Autodesk Fusion 360 part; units mm, degrees
note: some values were not read from the file. Set by a fixed rule: which sketch regions a step uses.
(part 20 of 20)
  spline S115 degree 5 poles (0.9213, 29.0307) (0.9213, 29.0307) (0.9213, 29.0309) (0.9213, 29.0313) (0.9213, 29.0318) (0.9213, 29.0325) (0.9213, 29.0334) (0.9214, 29.0344) (0.9214, 29.0355) (0.9214, 29.0367) (0.9214, 29.038) (0.9214, 29.0394) (0.9214, 29.0409) (0.9214, 29.0425) (0.9214, 29.0443) (0.9214, 29.0461) (0.9214, 29.0481) (0.9214, 29.0501) (0.9214, 29.0522) (0.9214, 29.0545) (0.9214, 29.0568) (0.9213, 29.0592) (0.9213, 29.0618) (0.9212, 29.0644) (0.9212, 29.0671) (0.9211, 29.0699) (0.9211, 29.0728) (0.921, 29.0758) (0.9209, 29.0788) (0.9208, 29.082) (0.9208, 29.0852) (0.9206, 29.0886) (0.9205, 29.092) (0.9204, 29.0955) (0.9203, 29.0991) (0.9201, 29.1028) (0.92, 29.1065) (0.9198, 29.1103) (0.9197, 29.1143) (0.9195, 29.1183) (0.9193, 29.1223) (0.9191, 29.1265) (0.9189, 29.1307) (0.9186, 29.135) (0.9184, 29.1394) (0.9182, 29.1439) (0.9179, 29.1484) (0.9176, 29.153) (0.9173, 29.1577) (0.917, 29.1624) (0.9167, 29.1673) (0.9164, 29.1722) (0.9161, 29.1771) (0.9157, 29.1822) (0.9153, 29.1873) (0.915, 29.1925) (0.9146, 29.1977) (0.9141, 29.203) (0.9137, 29.2084) (0.9133, 29.2139) (0.9128, 29.2194) (0.9124, 29.225) (0.9119, 29.2306) (0.9114, 29.2363) (0.9109, 29.2421) (0.9103, 29.248) (0.9098, 29.2539) (0.9092, 29.2599) (0.9087, 29.2659) (0.9081, 29.272) (0.9075, 29.2781) (0.9068, 29.2844) (0.9062, 29.2906) (0.9055, 29.297) (0.9049, 29.3034) (0.9042, 29.3099) (0.9035, 29.3164) (0.9027, 29.323) (0.902, 29.3296) (0.9012, 29.3363) (0.9005, 29.343) (0.8997, 29.3498) (0.8989, 29.3567) (0.898, 29.3636) (0.8972, 29.3706) (0.8963, 29.3777) (0.8954, 29.3847) (0.8945, 29.3919) (0.8936, 29.3991) (0.8927, 29.4063) (0.8917, 29.4137) (0.8907, 29.421) (0.8897, 29.4284) (0.8887, 29.4359) (0.8877, 29.4434) (0.8866, 29.451) (0.8856, 29.4586) (0.8845, 29.4663) (0.8834, 29.474) (0.8822, 29.4818) (0.8811, 29.4896) (0.8799, 29.4975) (0.8787, 29.5054) (0.8775, 29.5134) (0.8763, 29.5214) (0.875, 29.5295) (0.8738, 29.5376) (0.8725, 29.5458) (0.8712, 29.554) (0.8698, 29.5623) (0.8685, 29.5706) (0.8671, 29.5789) (0.8657, 29.5873) (0.8643, 29.5958) (0.8629, 29.6043) (0.8614, 29.6128) (0.86, 29.6214) (0.8585, 29.6301) (0.8569, 29.6388) (0.8554, 29.6475) (0.8538, 29.6563) (0.8523, 29.6651) (0.8507, 29.6739) (0.849, 29.6828) (0.8474, 29.6918) (0.8457, 29.7008) (0.844, 29.7098) (0.8423, 29.7189) (0.8406, 29.728) (0.8388, 29.7372) (0.8371, 29.7464) (0.8353, 29.7556) (0.8334, 29.7649) (0.8316, 29.7742) (0.8297, 29.7836) (0.8279, 29.793) (0.8259, 29.8025) (0.824, 29.812) (0.8221, 29.8215) (0.8201, 29.8311) (0.8181, 29.8407) (0.8161, 29.8503) (0.814, 29.86) (0.812, 29.8697) (0.8099, 29.8795) (0.8078, 29.8893) (0.8056, 29.8992) (0.8035, 29.909) (0.8013, 29.919) (0.7991, 29.9289) (0.7969, 29.9389) (0.7946, 29.949) (0.7923, 29.959) (0.79, 29.9691) (0.7877, 29.9793) (0.7854, 29.9895) (0.783, 29.9997) (0.7806, 30.0099) (0.7782, 30.0202) (0.7758, 30.0306) (0.7733, 30.0409) (0.7708, 30.0513) (0.7683, 30.0618) (0.7658, 30.0722) (0.7632, 30.0827) (0.7606, 30.0933) (0.758, 30.1038) (0.7554, 30.1145) (0.7528, 30.1251) (0.7501, 30.1358) (0.7474, 30.1465) (0.7447, 30.1572) (0.7419, 30.168) (0.7391, 30.1788) (0.7364, 30.1897) (0.7335, 30.2005) (0.7307, 30.2114) (0.7278, 30.2224) (0.7249, 30.2334) (0.722, 30.2444) (0.7191, 30.2554) (0.7161, 30.2665) (0.7131, 30.2776) (0.7101, 30.2887) (0.7071, 30.2999) (0.704, 30.3111) (0.7009, 30.3223) (0.6978, 30.3336) (0.6947, 30.3448) (0.6915, 30.3562) (0.6883, 30.3675) (0.6851, 30.3789) (0.6819, 30.3903) (0.6786, 30.4017) (0.6753, 30.4132) (0.672, 30.4247) (0.6687, 30.4362) (0.6653, 30.4478) (0.6619, 30.4594) (0.6585, 30.471) (0.6551, 30.4827) (0.6516, 30.4943) (0.6481, 30.506) (0.6446, 30.5178) (0.6411, 30.5295) (0.6375, 30.5413) (0.6339, 30.5531) (0.6303, 30.565) (0.6267, 30.5769) (0.623, 30.5888) (0.6193, 30.6007) (0.6156, 30.6126) (0.6118, 30.6246) (0.6081, 30.6366) (0.6043, 30.6487) (0.6005, 30.6607) (0.5966, 30.6728) (0.5927, 30.685) (0.5889, 30.6971) (0.5849, 30.7093) (0.581, 30.7215) (0.577, 30.7337) (0.573, 30.7459) (0.569, 30.7582) (0.5649, 30.7705) (0.5609, 30.7828) (0.5568, 30.7952) (0.5526, 30.8076) (0.5485, 30.82) (0.5443, 30.8324) (0.5401, 30.8448) (0.5359, 30.8573) (0.5316, 30.8698) (0.5273, 30.8823) (0.523, 30.8949) (0.5187, 30.9075) (0.5143, 30.9201) (0.5099, 30.9327) (0.5055, 30.9453) (0.5011, 30.958) (0.4966, 30.9707) (0.493, 30.9809) (0.4903, 30.9885) (0.4885, 30.9936) (0.4876, 30.9962) knots 0 0 0 0 0 0 0.00416667 0.00833333 0.0125 0.01666667 0.02083333 0.025 0.02916667 0.03333333 0.0375 0.04166667 0.04583333 0.05 0.05416667 0.05833333 0.0625 0.06666667 0.07083333 0.075 0.07916667 0.08333333 0.0875 0.09166667 0.09583333 0.1 0.10416667 0.10833333 0.1125 0.11666667 0.12083333 0.125 0.12916667 0.13333333 0.1375 0.14166667 0.14583333 0.15 0.15416667 0.15833333 0.1625 0.16666667 0.17083333 0.175 0.17916667 0.18333333 0.1875 0.19166667 0.19583333 0.2 0.20416667 0.20833333 0.2125 0.21666667 0.22083333 0.225 0.22916667 0.23333333 0.2375 0.24166667 0.24583333 0.25 0.25416667 0.25833333 0.2625 0.26666667 0.27083333 0.275 0.27916667 0.28333333 0.2875 0.29166667 0.29583333 0.3 0.30416667 0.30833333 0.3125 0.31666667 0.32083333 0.325 0.32916667 0.33333333 0.3375 0.34166667 0.34583333 0.35 0.35416667 0.35833333 0.3625 0.36666667 0.37083333 0.375 0.37916667 0.38333333 0.3875 0.39166667 0.39583333 0.4 0.40416667 0.40833333 0.4125 0.41666667 0.42083333 0.425 0.42916667 0.43333333 0.4375 0.44166667 0.44583333 0.45 0.45416667 0.45833333 0.4625 0.46666667 0.47083333 0.475 0.47916667 0.48333333 0.4875 0.49166667 0.49583333 0.5 0.50416667 0.50833333 0.5125 0.51666667 0.52083333 0.525 0.52916667 0.53333333 0.5375 0.54166667 0.54583333 0.55 0.55416667 0.55833333 0.5625 0.56666667 0.57083333 0.575 0.57916667 0.58333333 0.5875 0.59166667 0.59583333 0.6 0.60416667 0.60833333 0.6125 0.61666667 0.62083333 0.625 0.62916667 0.63333333 0.6375 0.64166667 0.64583333 0.65 0.65416667 0.65833333 0.6625 0.66666667 0.67083333 0.675 0.67916667 0.68333333 0.6875 0.69166667 0.69583333 0.7 0.70416667 0.70833333 0.7125 0.71666667 0.72083333 0.725 0.72916667 0.73333333 0.7375 0.74166667 0.74583333 0.75 0.75416667 0.75833333 0.7625 0.76666667 0.77083333 0.775 0.77916667 0.78333333 0.7875 0.79166667 0.79583333 0.8 0.80416667 0.80833333 0.8125 0.81666667 0.82083333 0.825 0.82916667 0.83333333 0.8375 0.84166667 0.84583333 0.85 0.85416667 0.85833333 0.8625 0.86666667 0.87083333 0.875 0.87916667 0.88333333 0.8875 0.89166667 0.89583333 0.9 0.90416667 0.90833333 0.9125 0.91666667 0.92083333 0.925 0.92916667 0.93333333 0.9375 0.94166667 0.94583333 0.95 0.95416667 0.95833333 0.9625 0.96666667 0.97083333 0.975 0.97916667 0.98333333 0.9875 0.99166667 0.99583333 1 1 1 1 1 1
  line L225 (-24.6799, 15.3128) -> (-24.6806, 15.3132)
  line L226 (0.9119, 28.7355) -> (0.9213, 29.0298)
  line L227 (0.9213, 29.0298) -> (0.9213, 29.0307)
  line L228 (-25.6019, 13.7175) -> (-25.6012, 13.7171)
  line L229 (-24.0271, 16.318) -> (-23.7836, 16.1526)
  arc A119 (2.0967, 28.6734) -> (0.9119, 28.7355) centre (0, 0) ccw
  arc A120 (-26.5997, 15.9204) -> (-27.0873, 15.0758) centre (0, 0) ccw
  line L230 (-27.8937, 8.0945) -> (-27.6109, 8.0125)
  arc A121 (-28.2972, 5.0824) -> (-28.4828, 3.9106) centre (0, 0) ccw
  spline S116 degree 5 poles (-28.2047, 6.937) (-28.2048, 6.937) (-28.205, 6.937) (-28.2053, 6.9371) (-28.2058, 6.9372) (-28.2065, 6.9374) (-28.2074, 6.9376) (-28.2083, 6.9378) (-28.2094, 6.9381) (-28.2106, 6.9383) (-28.2118, 6.9386) (-28.2132, 6.9389) (-28.2147, 6.9392) (-28.2163, 6.9396) (-28.218, 6.9399) (-28.2198, 6.9403) (-28.2217, 6.9407) (-28.2237, 6.9411) (-28.2258, 6.9416) (-28.228, 6.942) (-28.2303, 6.9425) (-28.2327, 6.9429) (-28.2351, 6.9434) (-28.2377, 6.9439) (-28.2404, 6.9445) (-28.2431, 6.945) (-28.246, 6.9455) (-28.2489, 6.9461) (-28.2519, 6.9466) (-28.255, 6.9472) (-28.2582, 6.9478) (-28.2615, 6.9484) (-28.2649, 6.949) (-28.2683, 6.9496) (-28.2719, 6.9502) (-28.2755, 6.9508) (-28.2792, 6.9515) (-28.283, 6.9521) (-28.2868, 6.9528) (-28.2908, 6.9534) (-28.2948, 6.9541) (-28.2989, 6.9547) (-28.3031, 6.9554) (-28.3074, 6.9561) (-28.3117, 6.9568) (-28.3161, 6.9574) (-28.3206, 6.9581) (-28.3252, 6.9588) (-28.3298, 6.9595) (-28.3345, 6.9602) (-28.3393, 6.9609) (-28.3442, 6.9616) (-28.3491, 6.9623) (-28.3541, 6.963) (-28.3592, 6.9637) (-28.3643, 6.9644) (-28.3695, 6.9651) (-28.3748, 6.9658) (-28.3802, 6.9665) (-28.3856, 6.9672) (-28.3911, 6.9679) (-28.3966, 6.9686) (-28.4023, 6.9693) (-28.408, 6.97) (-28.4137, 6.9707) (-28.4196, 6.9714) (-28.4255, 6.9721) (-28.4314, 6.9728) (-28.4374, 6.9735) (-28.4435, 6.9742) (-28.4497, 6.9749) (-28.4559, 6.9756) (-28.4622, 6.9763) (-28.4685, 6.9769) (-28.4749, 6.9776) (-28.4814, 6.9783) (-28.4879, 6.9789) (-28.4945, 6.9796) (-28.5011, 6.9803) (-28.5078, 6.9809) (-28.5146, 6.9816) (-28.5214, 6.9822) (-28.5283, 6.9828) (-28.5353, 6.9835) (-28.5423, 6.9841) (-28.5493, 6.9847) (-28.5564, 6.9853) (-28.5636, 6.9859) (-28.5709, 6.9865) (-28.5781, 6.9871) (-28.5855, 6.9877) (-28.5929, 6.9882) (-28.6004, 6.9888) (-28.6079, 6.9894) (-28.6154, 6.9899) (-28.6231, 6.9905) (-28.6307, 6.991) (-28.6385, 6.9915) (-28.6463, 6.9921) (-28.6541, 6.9926) (-28.662, 6.9931) (-28.67, 6.9936) (-28.678, 6.994) (-28.686, 6.9945) (-28.6941, 6.995) (-28.7023, 6.9954) (-28.7105, 6.9959) (-28.7187, 6.9963) (-28.727, 6.9968) (-28.7354, 6.9972) (-28.7438, 6.9976) (-28.7523, 6.998) (-28.7608, 6.9984) (-28.7694, 6.9987) (-28.778, 6.9991) (-28.7866, 6.9995) (-28.7953, 6.9998) (-28.8041, 7.0001) (-28.8129, 7.0005) (-28.8218, 7.0008) (-28.8307, 7.0011) (-28.8396, 7.0014) (-28.8486, 7.0016) (-28.8577, 7.0019) (-28.8668, 7.0021) (-28.8759, 7.0024) (-28.8851, 7.0026) (-28.8943, 7.0028) (-28.9036, 7.003) (-28.9129, 7.0032) (-28.9223, 7.0034) (-28.9317, 7.0036) (-28.9412, 7.0037) (-28.9507, 7.0038) (-28.9602, 7.004) (-28.9698, 7.0041) (-28.9795, 7.0042) (-28.9892, 7.0043) (-28.9989, 7.0043) (-29.0087, 7.0044) (-29.0185, 7.0044) (-29.0284, 7.0045) (-29.0383, 7.0045) (-29.0482, 7.0045) (-29.0582, 7.0045) (-29.0682, 7.0044) (-29.0783, 7.0044) (-29.0884, 7.0043) (-29.0986, 7.0043) (-29.1088, 7.0042) (-29.119, 7.0041) (-29.1293, 7.004) (-29.1396, 7.0038) (-29.15, 7.0037) (-29.1604, 7.0035) (-29.1708, 7.0034) (-29.1813, 7.0032) (-29.1919, 7.003) (-29.2024, 7.0028) (-29.213, 7.0025) (-29.2237, 7.0023) (-29.2344, 7.002) (-29.2451, 7.0017) (-29.2559, 7.0014) (-29.2667, 7.0011) (-29.2775, 7.0008) (-29.2884, 7.0004) (-29.2993, 7.0001) (-29.3103, 6.9997) (-29.3213, 6.9993) (-29.3323, 6.9989) (-29.3434, 6.9984) (-29.3545, 6.998) (-29.3657, 6.9975) (-29.3768, 6.997) (-29.3881, 6.9965) (-29.3993, 6.996) (-29.4106, 6.9955) (-29.422, 6.995) (-29.4333, 6.9944) (-29.4447, 6.9938) (-29.4562, 6.9932) (-29.4677, 6.9926) (-29.4792, 6.992) (-29.4907, 6.9913) (-29.5023, 6.9906) (-29.514, 6.99) (-29.5256, 6.9892) (-29.5373, 6.9885) (-29.549, 6.9878) (-29.5608, 6.987) (-29.5726, 6.9863) (-29.5844, 6.9855) (-29.5963, 6.9846) (-29.6082, 6.9838) (-29.6201, 6.983) (-29.6321, 6.9821) (-29.6441, 6.9812) (-29.6562, 6.9803) (-29.6682, 6.9794) (-29.6803, 6.9784) (-29.6925, 6.9775) (-29.7047, 6.9765) (-29.7169, 6.9755) (-29.7291, 6.9745) (-29.7414, 6.9735) (-29.7537, 6.9724) (-29.766, 6.9713) (-29.7784, 6.9702) (-29.7908, 6.9691) (-29.8032, 6.968) (-29.8157, 6.9669) (-29.8282, 6.9657) (-29.8407, 6.9645) (-29.8533, 6.9633) (-29.8659, 6.9621) (-29.8785, 6.9608) (-29.8912, 6.9596) (-29.9039, 6.9583) (-29.9166, 6.957) (-29.9293, 6.9556) (-29.9421, 6.9543) (-29.9549, 6.9529) (-29.9678, 6.9516) (-29.9806, 6.9501) (-29.9935, 6.9487) (-30.0065, 6.9473) (-30.0194, 6.9458) (-30.0324, 6.9443) (-30.0455, 6.9428) (-30.0585, 6.9413) (-30.0716, 6.9398) (-30.0847, 6.9382) (-30.0979, 6.9366) (-30.111, 6.935) (-30.1242, 6.9334) (-30.1375, 6.9317) (-30.1507, 6.9301) (-30.164, 6.9284) (-30.1773, 6.9267) (-30.1907, 6.925) (-30.2014, 6.9236) (-30.2094, 6.9225) (-30.2148, 6.9218) (-30.2174, 6.9214) knots 0 0 0 0 0 0 0.00416667 0.00833333 0.0125 0.01666667 0.02083333 0.025 0.02916667 0.03333333 0.0375 0.04166667 0.04583333 0.05 0.05416667 0.05833333 0.0625 0.06666667 0.07083333 0.075 0.07916667 0.08333333 0.0875 0.09166667 0.09583333 0.1 0.10416667 0.10833333 0.1125 0.11666667 0.12083333 0.125 0.12916667 0.13333333 0.1375 0.14166667 0.14583333 0.15 0.15416667 0.15833333 0.1625 0.16666667 0.17083333 0.175 0.17916667 0.18333333 0.1875 0.19166667 0.19583333 0.2 0.20416667 0.20833333 0.2125 0.21666667 0.22083333 0.225 0.22916667 0.23333333 0.2375 0.24166667 0.24583333 0.25 0.25416667 0.25833333 0.2625 0.26666667 0.27083333 0.275 0.27916667 0.28333333 0.2875 0.29166667 0.29583333 0.3 0.30416667 0.30833333 0.3125 0.31666667 0.32083333 0.325 0.32916667 0.33333333 0.3375 0.34166667 0.34583333 0.35 0.35416667 0.35833333 0.3625 0.36666667 0.37083333 0.375 0.37916667 0.38333333 0.3875 0.39166667 0.39583333 0.4 0.40416667 0.40833333 0.4125 0.41666667 0.42083333 0.425 0.42916667 0.43333333 0.4375 0.44166667 0.44583333 0.45 0.45416667 0.45833333 0.4625 0.46666667 0.47083333 0.475 0.47916667 0.48333333 0.4875 0.49166667 0.49583333 0.5 0.50416667 0.50833333 0.5125 0.51666667 0.52083333 0.525 0.52916667 0.53333333 0.5375 0.54166667 0.54583333 0.55 0.55416667 0.55833333 0.5625 0.56666667 0.57083333 0.575 0.57916667 0.58333333 0.5875 0.59166667 0.59583333 0.6 0.60416667 0.60833333 0.6125 0.61666667 0.62083333 0.625 0.62916667 0.63333333 0.6375 0.64166667 0.64583333 0.65 0.65416667 0.65833333 0.6625 0.66666667 0.67083333 0.675 0.67916667 0.68333333 0.6875 0.69166667 0.69583333 0.7 0.70416667 0.70833333 0.7125 0.71666667 0.72083333 0.725 0.72916667 0.73333333 0.7375 0.74166667 0.74583333 0.75 0.75416667 0.75833333 0.7625 0.76666667 0.77083333 0.775 0.77916667 0.78333333 0.7875 0.79166667 0.79583333 0.8 0.80416667 0.80833333 0.8125 0.81666667 0.82083333 0.825 0.82916667 0.83333333 0.8375 0.84166667 0.84583333 0.85 0.85416667 0.85833333 0.8625 0.86666667 0.87083333 0.875 0.87916667 0.88333333 0.8875 0.89166667 0.89583333 0.9 0.90416667 0.90833333 0.9125 0.91666667 0.92083333 0.925 0.92916667 0.93333333 0.9375 0.94166667 0.94583333 0.95 0.95416667 0.95833333 0.9625 0.96666667 0.97083333 0.975 0.97916667 0.98333333 0.9875 0.99166667 0.99583333 1 1 1 1 1 1
  line L231 (-28.587, 5.1345) -> (-28.2972, 5.0824)
  line L232 (-28.5878, 5.1346) -> (-28.587, 5.1345)
  spline S117 degree 5 poles (-30.4202, 5.9675) (-30.4179, 5.9661) (-30.4133, 5.9633) (-30.4064, 5.959) (-30.3972, 5.9534) (-30.3857, 5.9464) (-30.3742, 5.9394) (-30.3628, 5.9325) (-30.3513, 5.9255) (-30.3399, 5.9187) (-30.3285, 5.9118) (-30.3171, 5.905) (-30.3058, 5.8982) (-30.2944, 5.8914) (-30.2831, 5.8847) (-30.2718, 5.878) (-30.2605, 5.8713) (-30.2492, 5.8647) (-30.238, 5.8581) (-30.2268, 5.8515) (-30.2156, 5.8449) (-30.2044, 5.8384) (-30.1932, 5.8319) (-30.1821, 5.8255) (-30.1709, 5.8191) (-30.1598, 5.8127) (-30.1487, 5.8063) (-30.1377, 5.8) (-30.1266, 5.7937) (-30.1156, 5.7874) (-30.1046, 5.7811) (-30.0936, 5.7749) (-30.0826, 5.7688) (-30.0717, 5.7626) (-30.0608, 5.7565) (-30.0499, 5.7504) (-30.039, 5.7443) (-30.0281, 5.7383) (-30.0173, 5.7323) (-30.0065, 5.7263) (-29.9957, 5.7204) (-29.9849, 5.7145) (-29.9742, 5.7086) (-29.9634, 5.7028) (-29.9527, 5.697) (-29.9421, 5.6912) (-29.9314, 5.6854) (-29.9208, 5.6797) (-29.9102, 5.674) (-29.8996, 5.6683) (-29.889, 5.6627) (-29.8785, 5.6571) (-29.868, 5.6515) (-29.8575, 5.646) (-29.847, 5.6405) (-29.8366, 5.635) (-29.8262, 5.6296) (-29.8158, 5.6242) (-29.8054, 5.6188) (-29.7951, 5.6134) (-29.7847, 5.6081) (-29.7745, 5.6028) (-29.7642, 5.5975) (-29.754, 5.5923) (-29.7437, 5.5871) (-29.7336, 5.5819) (-29.7234, 5.5768) (-29.7133, 5.5717) (-29.7032, 5.5666) (-29.6931, 5.5615) (-29.683, 5.5565) (-29.673, 5.5515) (-29.663, 5.5466) (-29.653, 5.5416) (-29.6431, 5.5367) (-29.6332, 5.5319) (-29.6233, 5.527) (-29.6134, 5.5222) (-29.6036, 5.5175) (-29.5938, 5.5127) (-29.584, 5.508) (-29.5743, 5.5033) (-29.5646, 5.4987) (-29.5549, 5.494) (-29.5452, 5.4895) (-29.5356, 5.4849) (-29.526, 5.4804) (-29.5165, 5.4759) (-29.5069, 5.4714) (-29.4974, 5.467) (-29.4879, 5.4625) (-29.4785, 5.4582) (-29.4691, 5.4538) (-29.4597, 5.4495) (-29.4504, 5.4452) (-29.441, 5.441) (-29.4318, 5.4367) (-29.4225, 5.4325) (-29.4133, 5.4284) (-29.4041, 5.4242) (-29.395, 5.4201) (-29.3858, 5.4161) (-29.3767, 5.412) (-29.3677, 5.408) (-29.3587, 5.404) (-29.3497, 5.4001) (-29.3407, 5.3961) (-29.3318, 5.3922) (-29.3229, 5.3884) (-29.3141, 5.3846) (-29.3053, 5.3807) (-29.2965, 5.377) (-29.2878, 5.3732) (-29.279, 5.3695) (-29.2704, 5.3658) (-29.2617, 5.3622) (-29.2531, 5.3586) (-29.2446, 5.355) (-29.2361, 5.3514) (-29.2276, 5.3479) (-29.2191, 5.3444) (-29.2107, 5.3409) (-29.2023, 5.3375) (-29.194, 5.3341) (-29.1857, 5.3307) (-29.1775, 5.3273) (-29.1692, 5.324) (-29.1611, 5.3207) (-29.1529, 5.3175) (-29.1448, 5.3143) (-29.1368, 5.3111) (-29.1288, 5.3079) (-29.1208, 5.3047) (-29.1129, 5.3016) (-29.105, 5.2986) (-29.0971, 5.2955) (-29.0893, 5.2925) (-29.0815, 5.2895) (-29.0738, 5.2865) (-29.0661, 5.2836) (-29.0585, 5.2807) (-29.0509, 5.2778) (-29.0433, 5.275) (-29.0358, 5.2722) (-29.0284, 5.2694) (-29.021, 5.2666) (-29.0136, 5.2639) (-29.0063, 5.2612) (-28.999, 5.2586) (-28.9918, 5.2559) (-28.9846, 5.2533) (-28.9774, 5.2508) (-28.9703, 5.2482) (-28.9633, 5.2457) (-28.9563, 5.2432) (-28.9493, 5.2408) (-28.9424, 5.2383) (-28.9356, 5.2359) (-28.9288, 5.2336) (-28.922, 5.2312) (-28.9153, 5.2289) (-28.9087, 5.2266) (-28.9021, 5.2244) (-28.8955, 5.2222) (-28.889, 5.22) (-28.8826, 5.2178) (-28.8762, 5.2157) (-28.8699, 5.2136) (-28.8636, 5.2115) (-28.8573, 5.2094) (-28.8512, 5.2074) (-28.8451, 5.2054) (-28.839, 5.2035) (-28.833, 5.2015) (-28.827, 5.1996) (-28.8211, 5.1978) (-28.8153, 5.1959) (-28.8095, 5.1941) (-28.8038, 5.1923) (-28.7981, 5.1905) (-28.7925, 5.1888) (-28.7869, 5.1871) (-28.7815, 5.1854) (-28.776, 5.1838) (-28.7707, 5.1822) (-28.7654, 5.1806) (-28.7601, 5.179) (-28.7549, 5.1775) (-28.7498, 5.176) (-28.7448, 5.1745) (-28.7398, 5.173) (-28.7349, 5.1716) (-28.73, 5.1702) (-28.7252, 5.1689) (-28.7205, 5.1675) (-28.7158, 5.1662) (-28.7112, 5.1649) (-28.7067, 5.1637) (-28.7023, 5.1625) (-28.6979, 5.1613) (-28.6936, 5.1601) (-28.6893, 5.1589) (-28.6852, 5.1578) (-28.6811, 5.1567) (-28.6771, 5.1557) (-28.6731, 5.1546) (-28.6693, 5.1536) (-28.6655, 5.1527) (-28.6617, 5.1517) (-28.6581, 5.1508) (-28.6545, 5.1499) (-28.6511, 5.149) (-28.6477, 5.1481) (-28.6443, 5.1473) (-28.6411, 5.1465) (-28.6379, 5.1458) (-28.6349, 5.145) (-28.6319, 5.1443) (-28.629, 5.1436) (-28.6262, 5.143) (-28.6234, 5.1423) (-28.6208, 5.1417) (-28.6182, 5.1411) (-28.6158, 5.1406) (-28.6134, 5.14) (-28.6111, 5.1395) (-28.6089, 5.139) (-28.6069, 5.1386) (-28.6049, 5.1381) (-28.603, 5.1377) (-28.6012, 5.1374) (-28.5995, 5.137) (-28.5979, 5.1367) (-28.5964, 5.1363) (-28.595, 5.1361) (-28.5937, 5.1358) (-28.5925, 5.1356) (-28.5915, 5.1354) (-28.5905, 5.1352) (-28.5896, 5.135) (-28.5889, 5.1349) (-28.5884, 5.1348) (-28.5881, 5.1347) (-28.5879, 5.1347) (-28.5878, 5.1346) knots -1 -1 -1 -1 -1 -1 -0.99583333 -0.99166667 -0.9875 -0.98333333 -0.97916667 -0.975 -0.97083333 -0.96666667 -0.9625 -0.95833333 -0.95416667 -0.95 -0.94583333 -0.94166667 -0.9375 -0.93333333 -0.92916667 -0.925 -0.92083333 -0.91666667 -0.9125 -0.90833333 -0.90416667 -0.9 -0.89583333 -0.89166667 -0.8875 -0.88333333 -0.87916667 -0.875 -0.87083333 -0.86666667 -0.8625 -0.85833333 -0.85416667 -0.85 -0.84583333 -0.84166667 -0.8375 -0.83333333 -0.82916667 -0.825 -0.82083333 -0.81666667 -0.8125 -0.80833333 -0.80416667 -0.8 -0.79583333 -0.79166667 -0.7875 -0.78333333 -0.77916667 -0.775 -0.77083333 -0.76666667 -0.7625 -0.75833333 -0.75416667 -0.75 -0.74583333 -0.74166667 -0.7375 -0.73333333 -0.72916667 -0.725 -0.72083333 -0.71666667 -0.7125 -0.70833333 -0.70416667 -0.7 -0.69583333 -0.69166667 -0.6875 -0.68333333 -0.67916667 -0.675 -0.67083333 -0.66666667 -0.6625 -0.65833333 -0.65416667 -0.65 -0.64583333 -0.64166667 -0.6375 -0.63333333 -0.62916667 -0.625 -0.62083333 -0.61666667 -0.6125 -0.60833333 -0.60416667 -0.6 -0.59583333 -0.59166667 -0.5875 -0.58333333 -0.57916667 -0.575 -0.57083333 -0.56666667 -0.5625 -0.55833333 -0.55416667 -0.55 -0.54583333 -0.54166667 -0.5375 -0.53333333 -0.52916667 -0.525 -0.52083333 -0.51666667 -0.5125 -0.50833333 -0.50416667 -0.5 -0.49583333 -0.49166667 -0.4875 -0.48333333 -0.47916667 -0.475 -0.47083333 -0.46666667 -0.4625 -0.45833333 -0.45416667 -0.45 -0.44583333 -0.44166667 -0.4375 -0.43333333 -0.42916667 -0.425 -0.42083333 -0.41666667 -0.4125 -0.40833333 -0.40416667 -0.4 -0.39583333 -0.39166667 -0.3875 -0.38333333 -0.37916667 -0.375 -0.37083333 -0.36666667 -0.3625 -0.35833333 -0.35416667 -0.35 -0.34583333 -0.34166667 -0.3375 -0.33333333 -0.32916667 -0.325 -0.32083333 -0.31666667 -0.3125 -0.30833333 -0.30416667 -0.3 -0.29583333 -0.29166667 -0.2875 -0.28333333 -0.27916667 -0.275 -0.27083333 -0.26666667 -0.2625 -0.25833333 -0.25416667 -0.25 -0.24583333 -0.24166667 -0.2375 -0.23333333 -0.22916667 -0.225 -0.22083333 -0.21666667 -0.2125 -0.20833333 -0.20416667 -0.2 -0.19583333 -0.19166667 -0.1875 -0.18333333 -0.17916667 -0.175 -0.17083333 -0.16666667 -0.1625 -0.15833333 -0.15416667 -0.15 -0.14583333 -0.14166667 -0.1375 -0.13333333 -0.12916667 -0.125 -0.12083333 -0.11666667 -0.1125 -0.10833333 -0.10416667 -0.1 -0.09583333 -0.09166667 -0.0875 -0.08333333 -0.07916667 -0.075 -0.07083333 -0.06666667 -0.0625 -0.05833333 -0.05416667 -0.05 -0.04583333 -0.04166667 -0.0375 -0.03333333 -0.02916667 -0.025 -0.02083333 -0.01666667 -0.0125 -0.00833333 -0.00416667 0 0 0 0 0 0
  arc A122 (-30.2174, 6.9214) -> (-30.4202, 5.9675) centre (0, 0) ccw
  line L233 (8.0945, 27.8937) -> (8.0125, 27.6109)
  line L234 (8.0948, 27.8945) -> (8.0945, 27.8937)
  line L235 (6.8665, 27.918) -> (6.9368, 28.2039)
  line L236 (-28.2039, 6.9368) -> (-28.2047, 6.937)
  line L237 (-27.918, 6.8665) -> (-28.2039, 6.9368)
  line L238 (-27.3243, 9.8469) -> (-27.3251, 9.8472)
  line L239 (-27.0473, 9.7471) -> (-27.3243, 9.8469)
  arc A123 (-26.6221, 10.8547) -> (-27.0473, 9.7471) centre (0, 0) ccw
  spline S118 degree 5 poles (5.9675, 30.4202) (5.9661, 30.4179) (5.9633, 30.4133) (5.959, 30.4064) (5.9534, 30.3972) (5.9464, 30.3857) (5.9394, 30.3742) (5.9325, 30.3628) (5.9255, 30.3513) (5.9187, 30.3399) (5.9118, 30.3285) (5.905, 30.3171) (5.8982, 30.3058) (5.8914, 30.2944) (5.8847, 30.2831) (5.878, 30.2718) (5.8713, 30.2605) (5.8647, 30.2492) (5.8581, 30.238) (5.8515, 30.2268) (5.8449, 30.2156) (5.8384, 30.2044) (5.8319, 30.1932) (5.8255, 30.1821) (5.8191, 30.1709) (5.8127, 30.1598) (5.8063, 30.1487) (5.8, 30.1377) (5.7937, 30.1266) (5.7874, 30.1156) (5.7811, 30.1046) (5.7749, 30.0936) (5.7688, 30.0826) (5.7626, 30.0717) (5.7565, 30.0608) (5.7504, 30.0499) (5.7443, 30.039) (5.7383, 30.0281) (5.7323, 30.0173) (5.7263, 30.0065) (5.7204, 29.9957) (5.7145, 29.9849) (5.7086, 29.9742) (5.7028, 29.9634) (5.697, 29.9527) (5.6912, 29.9421) (5.6854, 29.9314) (5.6797, 29.9208) (5.674, 29.9102) (5.6683, 29.8996) (5.6627, 29.889) (5.6571, 29.8785) (5.6515, 29.868) (5.646, 29.8575) (5.6405, 29.847) (5.635, 29.8366) (5.6296, 29.8262) (5.6242, 29.8158) (5.6188, 29.8054) (5.6134, 29.7951) (5.6081, 29.7847) (5.6028, 29.7745) (5.5975, 29.7642) (5.5923, 29.754) (5.5871, 29.7437) (5.5819, 29.7336) (5.5768, 29.7234) (5.5717, 29.7133) (5.5666, 29.7032) (5.5615, 29.6931) (5.5565, 29.683) (5.5515, 29.673) (5.5466, 29.663) (5.5416, 29.653) (5.5367, 29.6431) (5.5319, 29.6332) (5.527, 29.6233) (5.5222, 29.6134) (5.5175, 29.6036) (5.5127, 29.5938) (5.508, 29.584) (5.5033, 29.5743) (5.4987, 29.5646) (5.494, 29.5549) (5.4895, 29.5452) (5.4849, 29.5356) (5.4804, 29.526) (5.4759, 29.5165) (5.4714, 29.5069) (5.467, 29.4974) (5.4625, 29.4879) (5.4582, 29.4785) (5.4538, 29.4691) (5.4495, 29.4597) (5.4452, 29.4504) (5.441, 29.441) (5.4367, 29.4318) (5.4325, 29.4225) (5.4284, 29.4133) (5.4242, 29.4041) (5.4201, 29.395) (5.4161, 29.3858) (5.412, 29.3767) (5.408, 29.3677) (5.404, 29.3587) (5.4001, 29.3497) (5.3961, 29.3407) (5.3922, 29.3318) (5.3884, 29.3229) (5.3846, 29.3141) (5.3807, 29.3053) (5.377, 29.2965) (5.3732, 29.2878) (5.3695, 29.279) (5.3658, 29.2704) (5.3622, 29.2617) (5.3586, 29.2531) (5.355, 29.2446) (5.3514, 29.2361) (5.3479, 29.2276) (5.3444, 29.2191) (5.3409, 29.2107) (5.3375, 29.2023) (5.3341, 29.194) (5.3307, 29.1857) (5.3273, 29.1775) (5.324, 29.1692) (5.3207, 29.1611) (5.3175, 29.1529) (5.3143, 29.1448) (5.3111, 29.1368) (5.3079, 29.1288) (5.3047, 29.1208) (5.3016, 29.1129) (5.2986, 29.105) (5.2955, 29.0971) (5.2925, 29.0893) (5.2895, 29.0815) (5.2865, 29.0738) (5.2836, 29.0661) (5.2807, 29.0585) (5.2778, 29.0509) (5.275, 29.0433) (5.2722, 29.0358) (5.2694, 29.0284) (5.2666, 29.021) (5.2639, 29.0136) (5.2612, 29.0063) (5.2586, 28.999) (5.2559, 28.9918) (5.2533, 28.9846) (5.2508, 28.9774) (5.2482, 28.9703) (5.2457, 28.9633) (5.2432, 28.9563) (5.2408, 28.9493) (5.2383, 28.9424) (5.2359, 28.9356) (5.2336, 28.9288) (5.2312, 28.922) (5.2289, 28.9153) (5.2266, 28.9087) (5.2244, 28.9021) (5.2222, 28.8955) (5.22, 28.889) (5.2178, 28.8826) (5.2157, 28.8762) (5.2136, 28.8699) (5.2115, 28.8636) (5.2094, 28.8573) (5.2074, 28.8512) (5.2054, 28.8451) (5.2035, 28.839) (5.2015, 28.833) (5.1996, 28.827) (5.1978, 28.8211) (5.1959, 28.8153) (5.1941, 28.8095) (5.1923, 28.8038) (5.1905, 28.7981) (5.1888, 28.7925) (5.1871, 28.7869) (5.1854, 28.7815) (5.1838, 28.776) (5.1822, 28.7707) (5.1806, 28.7654) (5.179, 28.7601) (5.1775, 28.7549) (5.176, 28.7498) (5.1745, 28.7448) (5.173, 28.7398) (5.1716, 28.7349) (5.1702, 28.73) (5.1689, 28.7252) (5.1675, 28.7205) (5.1662, 28.7158) (5.1649, 28.7112) (5.1637, 28.7067) (5.1625, 28.7023) (5.1613, 28.6979) (5.1601, 28.6936) (5.1589, 28.6893) (5.1578, 28.6852) (5.1567, 28.6811) (5.1557, 28.6771) (5.1546, 28.6731) (5.1536, 28.6693) (5.1527, 28.6655) (5.1517, 28.6617) (5.1508, 28.6581) (5.1499, 28.6545) (5.149, 28.6511) (5.1481, 28.6477) (5.1473, 28.6443) (5.1465, 28.6411) (5.1458, 28.6379) (5.145, 28.6349) (5.1443, 28.6319) (5.1436, 28.629) (5.143, 28.6262) (5.1423, 28.6234) (5.1417, 28.6208) (5.1411, 28.6182) (5.1406, 28.6158) (5.14, 28.6134) (5.1395, 28.6111) (5.139, 28.6089) (5.1386, 28.6069) (5.1381, 28.6049) (5.1377, 28.603) (5.1374, 28.6012) (5.137, 28.5995) (5.1367, 28.5979) (5.1363, 28.5964) (5.1361, 28.595) (5.1358, 28.5937) (5.1356, 28.5925) (5.1354, 28.5915) (5.1352, 28.5905) (5.135, 28.5896) (5.1349, 28.5889) (5.1348, 28.5884) (5.1347, 28.5881) (5.1347, 28.5879) (5.1346, 28.5878) knots -1 -1 -1 -1 -1 -1 -0.99583333 -0.99166667 -0.9875 -0.98333333 -0.97916667 -0.975 -0.97083333 -0.96666667 -0.9625 -0.95833333 -0.95416667 -0.95 -0.94583333 -0.94166667 -0.9375 -0.93333333 -0.92916667 -0.925 -0.92083333 -0.91666667 -0.9125 -0.90833333 -0.90416667 -0.9 -0.89583333 -0.89166667 -0.8875 -0.88333333 -0.87916667 -0.875 -0.87083333 -0.86666667 -0.8625 -0.85833333 -0.85416667 -0.85 -0.84583333 -0.84166667 -0.8375 -0.83333333 -0.82916667 -0.825 -0.82083333 -0.81666667 -0.8125 -0.80833333 -0.80416667 -0.8 -0.79583333 -0.79166667 -0.7875 -0.78333333 -0.77916667 -0.775 -0.77083333 -0.76666667 -0.7625 -0.75833333 -0.75416667 -0.75 -0.74583333 -0.74166667 -0.7375 -0.73333333 -0.72916667 -0.725 -0.72083333 -0.71666667 -0.7125 -0.70833333 -0.70416667 -0.7 -0.69583333 -0.69166667 -0.6875 -0.68333333 -0.67916667 -0.675 -0.67083333 -0.66666667 -0.6625 -0.65833333 -0.65416667 -0.65 -0.64583333 -0.64166667 -0.6375 -0.63333333 -0.62916667 -0.625 -0.62083333 -0.61666667 -0.6125 -0.60833333 -0.60416667 -0.6 -0.59583333 -0.59166667 -0.5875 -0.58333333 -0.57916667 -0.575 -0.57083333 -0.56666667 -0.5625 -0.55833333 -0.55416667 -0.55 -0.54583333 -0.54166667 -0.5375 -0.53333333 -0.52916667 -0.525 -0.52083333 -0.51666667 -0.5125 -0.50833333 -0.50416667 -0.5 -0.49583333 -0.49166667 -0.4875 -0.48333333 -0.47916667 -0.475 -0.47083333 -0.46666667 -0.4625 -0.45833333 -0.45416667 -0.45 -0.44583333 -0.44166667 -0.4375 -0.43333333 -0.42916667 -0.425 -0.42083333 -0.41666667 -0.4125 -0.40833333 -0.40416667 -0.4 -0.39583333 -0.39166667 -0.3875 -0.38333333 -0.37916667 -0.375 -0.37083333 -0.36666667 -0.3625 -0.35833333 -0.35416667 -0.35 -0.34583333 -0.34166667 -0.3375 -0.33333333 -0.32916667 -0.325 -0.32083333 -0.31666667 -0.3125 -0.30833333 -0.30416667 -0.3 -0.29583333 -0.29166667 -0.2875 -0.28333333 -0.27916667 -0.275 -0.27083333 -0.26666667 -0.2625 -0.25833333 -0.25416667 -0.25 -0.24583333 -0.24166667 -0.2375 -0.23333333 -0.22916667 -0.225 -0.22083333 -0.21666667 -0.2125 -0.20833333 -0.20416667 -0.2 -0.19583333 -0.19166667 -0.1875 -0.18333333 -0.17916667 -0.175 -0.17083333 -0.16666667 -0.1625 -0.15833333 -0.15416667 -0.15 -0.14583333 -0.14166667 -0.1375 -0.13333333 -0.12916667 -0.125 -0.12083333 -0.11666667 -0.1125 -0.10833333 -0.10416667 -0.1 -0.09583333 -0.09166667 -0.0875 -0.08333333 -0.07916667 -0.075 -0.07083333 -0.06666667 -0.0625 -0.05833333 -0.05416667 -0.05 -0.04583333 -0.04166667 -0.0375 -0.03333333 -0.02916667 -0.025 -0.02083333 -0.01666667 -0.0125 -0.00833333 -0.00416667 0 0 0 0 0 0
  spline S119 degree 5 poles (-27.3251, 9.8472) (-27.3252, 9.8472) (-27.3254, 9.8473) (-27.3257, 9.8474) (-27.3262, 9.8475) (-27.3269, 9.8478) (-27.3277, 9.8481) (-27.3286, 9.8484) (-27.3296, 9.8487) (-27.3308, 9.8491) (-27.332, 9.8495) (-27.3334, 9.85) (-27.3348, 9.8505) (-27.3364, 9.851) (-27.338, 9.8515) (-27.3398, 9.8521) (-27.3416, 9.8527) (-27.3435, 9.8533) (-27.3456, 9.8539) (-27.3477, 9.8546) (-27.3499, 9.8553) (-27.3523, 9.856) (-27.3547, 9.8568) (-27.3572, 9.8575) (-27.3598, 9.8583) (-27.3625, 9.8591) (-27.3652, 9.86) (-27.3681, 9.8608) (-27.371, 9.8617) (-27.3741, 9.8626) (-27.3772, 9.8635) (-27.3804, 9.8645) (-27.3837, 9.8654) (-27.387, 9.8664) (-27.3905, 9.8674) (-27.394, 9.8684) (-27.3976, 9.8694) (-27.4013, 9.8704) (-27.4051, 9.8715) (-27.409, 9.8725) (-27.4129, 9.8736) (-27.4169, 9.8747) (-27.421, 9.8758) (-27.4252, 9.8769) (-27.4294, 9.878) (-27.4337, 9.8792) (-27.4381, 9.8803) (-27.4426, 9.8815) (-27.4471, 9.8827) (-27.4517, 9.8838) (-27.4564, 9.885) (-27.4612, 9.8862) (-27.466, 9.8874) (-27.4709, 9.8887) (-27.4759, 9.8899) (-27.481, 9.8911) (-27.4861, 9.8924) (-27.4912, 9.8936) (-27.4965, 9.8949) (-27.5018, 9.8962) (-27.5072, 9.8974) (-27.5127, 9.8987) (-27.5182, 9.9) (-27.5238, 9.9013) (-27.5294, 9.9026) (-27.5352, 9.9039) (-27.5409, 9.9052) (-27.5468, 9.9065) (-27.5527, 9.9079) (-27.5587, 9.9092) (-27.5647, 9.9105) (-27.5709, 9.9118) (-27.577, 9.9132) (-27.5833, 9.9145) (-27.5896, 9.9158) (-27.5959, 9.9172) (-27.6023, 9.9185) (-27.6088, 9.9199) (-27.6154, 9.9212) (-27.622, 9.9225) (-27.6286, 9.9239) (-27.6353, 9.9252) (-27.6421, 9.9266) (-27.649, 9.9279) (-27.6559, 9.9293) (-27.6628, 9.9306) (-27.6698, 9.932) (-27.6769, 9.9333) (-27.6841, 9.9347) (-27.6912, 9.936) (-27.6985, 9.9374) (-27.7058, 9.9387) (-27.7132, 9.9401) (-27.7206, 9.9414) (-27.728, 9.9428) (-27.7356, 9.9441) (-27.7431, 9.9454) (-27.7508, 9.9468) (-27.7585, 9.9481) (-27.7662, 9.9494) (-27.774, 9.9508) (-27.7819, 9.9521) (-27.7898, 9.9534) (-27.7977, 9.9547) (-27.8057, 9.956) (-27.8138, 9.9573) (-27.8219, 9.9586) (-27.8301, 9.9599) (-27.8383, 9.9612) (-27.8466, 9.9625) (-27.8549, 9.9638) (-27.8633, 9.9651) (-27.8717, 9.9664) (-27.8802, 9.9676) (-27.8887, 9.9689) (-27.8973, 9.9701) (-27.9059, 9.9714) (-27.9146, 9.9726) (-27.9233, 9.9739) (-27.9321, 9.9751) (-27.9409, 9.9763) (-27.9498, 9.9776) (-27.9587, 9.9788) (-27.9677, 9.98) (-27.9767, 9.9812) (-27.9858, 9.9824) (-27.9949, 9.9836) (-28.004, 9.9847) (-28.0133, 9.9859) (-28.0225, 9.9871) (-28.0318, 9.9882) (-28.0412, 9.9894) (-28.0506, 9.9905) (-28.06, 9.9916) (-28.0695, 9.9928) (-28.079, 9.9939) (-28.0886, 9.995) (-28.0982, 9.9961) (-28.1079, 9.9972) (-28.1176, 9.9983) (-28.1274, 9.9993) (-28.1372, 10.0004) (-28.147, 10.0014) (-28.1569, 10.0025) (-28.1668, 10.0035) (-28.1768, 10.0045) (-28.1868, 10.0055) (-28.1969, 10.0065) (-28.207, 10.0075) (-28.2172, 10.0085) (-28.2274, 10.0095) (-28.2376, 10.0104) (-28.2479, 10.0114) (-28.2582, 10.0123) (-28.2686, 10.0133) (-28.279, 10.0142) (-28.2894, 10.0151) (-28.2999, 10.016) (-28.3105, 10.0169) (-28.321, 10.0177) (-28.3317, 10.0186) (-28.3423, 10.0195) (-28.353, 10.0203) (-28.3638, 10.0211) (-28.3745, 10.0219) (-28.3854, 10.0227) (-28.3962, 10.0235) (-28.4071, 10.0243) (-28.4181, 10.0251) (-28.429, 10.0258) (-28.44, 10.0266) (-28.4511, 10.0273) (-28.4622, 10.028) (-28.4733, 10.0287) (-28.4845, 10.0294) (-28.4957, 10.0301) (-28.507, 10.0308) (-28.5183, 10.0314) (-28.5296, 10.0321) (-28.541, 10.0327) (-28.5524, 10.0333) (-28.5638, 10.0339) (-28.5753, 10.0345) (-28.5868, 10.0351) (-28.5984, 10.0356) (-28.61, 10.0362) (-28.6216, 10.0367) (-28.6333, 10.0372) (-28.645, 10.0377) (-28.6567, 10.0382) (-28.6685, 10.0387) (-28.6803, 10.0392) (-28.6922, 10.0396) (-28.7041, 10.04) (-28.716, 10.0405) (-28.728, 10.0409) (-28.74, 10.0412) (-28.752, 10.0416) (-28.7641, 10.042) (-28.7762, 10.0423) (-28.7883, 10.0427) (-28.8005, 10.043) (-28.8127, 10.0433) (-28.8249, 10.0436) (-28.8372, 10.0438) (-28.8495, 10.0441) (-28.8619, 10.0443) (-28.8743, 10.0445) (-28.8867, 10.0448) (-28.8991, 10.0449) (-28.9116, 10.0451) (-28.9241, 10.0453) (-28.9367, 10.0454) (-28.9493, 10.0456) (-28.9619, 10.0457) (-28.9745, 10.0458) (-28.9872, 10.0458) (-29, 10.0459) (-29.0127, 10.046) (-29.0255, 10.046) (-29.0383, 10.046) (-29.0512, 10.046) (-29.0641, 10.046) (-29.077, 10.046) (-29.0899, 10.0459) (-29.1029, 10.0458) (-29.1159, 10.0458) (-29.129, 10.0457) (-29.142, 10.0455) (-29.1551, 10.0454) (-29.1683, 10.0453) (-29.1815, 10.0451) (-29.1947, 10.0449) (-29.2079, 10.0447) (-29.2212, 10.0445) (-29.2345, 10.0442) (-29.2478, 10.044) (-29.2612, 10.0437) (-29.2745, 10.0434) (-29.288, 10.0431) (-29.3014, 10.0428) (-29.3122, 10.0425) (-29.3203, 10.0423) (-29.3257, 10.0422) (-29.3284, 10.0421) knots 0 0 0 0 0 0 0.00416667 0.00833333 0.0125 0.01666667 0.02083333 0.025 0.02916667 0.03333333 0.0375 0.04166667 0.04583333 0.05 0.05416667 0.05833333 0.0625 0.06666667 0.07083333 0.075 0.07916667 0.08333333 0.0875 0.09166667 0.09583333 0.1 0.10416667 0.10833333 0.1125 0.11666667 0.12083333 0.125 0.12916667 0.13333333 0.1375 0.14166667 0.14583333 0.15 0.15416667 0.15833333 0.1625 0.16666667 0.17083333 0.175 0.17916667 0.18333333 0.1875 0.19166667 0.19583333 0.2 0.20416667 0.20833333 0.2125 0.21666667 0.22083333 0.225 0.22916667 0.23333333 0.2375 0.24166667 0.24583333 0.25 0.25416667 0.25833333 0.2625 0.26666667 0.27083333 0.275 0.27916667 0.28333333 0.2875 0.29166667 0.29583333 0.3 0.30416667 0.30833333 0.3125 0.31666667 0.32083333 0.325 0.32916667 0.33333333 0.3375 0.34166667 0.34583333 0.35 0.35416667 0.35833333 0.3625 0.36666667 0.37083333 0.375 0.37916667 0.38333333 0.3875 0.39166667 0.39583333 0.4 0.40416667 0.40833333 0.4125 0.41666667 0.42083333 0.425 0.42916667 0.43333333 0.4375 0.44166667 0.44583333 0.45 0.45416667 0.45833333 0.4625 0.46666667 0.47083333 0.475 0.47916667 0.48333333 0.4875 0.49166667 0.49583333 0.5 0.50416667 0.50833333 0.5125 0.51666667 0.52083333 0.525 0.52916667 0.53333333 0.5375 0.54166667 0.54583333 0.55 0.55416667 0.55833333 0.5625 0.56666667 0.57083333 0.575 0.57916667 0.58333333 0.5875 0.59166667 0.59583333 0.6 0.60416667 0.60833333 0.6125 0.61666667 0.62083333 0.625 0.62916667 0.63333333 0.6375 0.64166667 0.64583333 0.65 0.65416667 0.65833333 0.6625 0.66666667 0.67083333 0.675 0.67916667 0.68333333 0.6875 0.69166667 0.69583333 0.7 0.70416667 0.70833333 0.7125 0.71666667 0.72083333 0.725 0.72916667 0.73333333 0.7375 0.74166667 0.74583333 0.75 0.75416667 0.75833333 0.7625 0.76666667 0.77083333 0.775 0.77916667 0.78333333 0.7875 0.79166667 0.79583333 0.8 0.80416667 0.80833333 0.8125 0.81666667 0.82083333 0.825 0.82916667 0.83333333 0.8375 0.84166667 0.84583333 0.85 0.85416667 0.85833333 0.8625 0.86666667 0.87083333 0.875 0.87916667 0.88333333 0.8875 0.89166667 0.89583333 0.9 0.90416667 0.90833333 0.9125 0.91666667 0.92083333 0.925 0.92916667 0.93333333 0.9375 0.94166667 0.94583333 0.95 0.95416667 0.95833333 0.9625 0.96666667 0.97083333 0.975 0.97916667 0.98333333 0.9875 0.99166667 0.99583333 1 1 1 1 1 1
  arc A124 (-29.3284, 10.0421) -> (-29.6298, 9.1146) centre (0, 0) ccw
extrude "押し出し1" add sketch "スケッチ1" along normal blind 3
